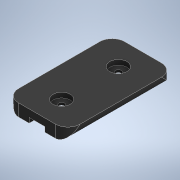
# Autodesk Inventor part: Gripper 5-4
Saved by Autodesk Inventor 2021 (Build 250183000, 183)
## iProperties
Created: 2022-01-10
Part Number: Gripper 5-4
Material: Generic
Document SubType Name: Modeling
Designer: Łukasz
Density: 1 g/cm^3
Appearance: Rubber - Black
Author: Łukasz
Autodesk Inventor part; units mm, degrees
ref_plane "YZ Plane" through (0, 0, 0) normal (1, 0, 0) x (0, 1, 0)
ref_plane "XZ Plane" through (0, 0, 0) normal (0, 1, 0) x (-1, 0, 0)
ref_plane "XY Plane" through (0, 0, 0) normal (0, 0, 1) x (1, 0, 0)
sketch "Sketch1" plane through (0, 0, 0) normal (0, 0, 1) x (1, 0, 0)
  line L0 (0, 2) -> (3.2, 2)
  line L1 (3.2, 2) -> (3.2, 0)
  line L2 (3.2, 0) -> (12.5, 0)
  line L3 (12.5, 0) -> (12.5, 5)
  line L4 (12.5, 5) -> (0, 5)
  line L5 (0, 0) -> (0, 5) construction
  line L6 (0, 2) -> (-3.2, 2)
  line L7 (-3.2, 2) -> (-3.2, 0)
  line L8 (-3.2, 0) -> (-12.5, 0)
  line L9 (-12.5, 0) -> (-12.5, 5)
  line L10 (-12.5, 5) -> (0, 5)
  dimension "d0" = 3.2
  dimension "d1" = 2
  dimension "d2" = 9.3
  dimension "d3" = 5
  constraints: 22 end point, 4 perpendicular, 4 symmetric about line, 1 horizontal, 1 vertical
  measures "d0" distance of L0.start L0.end
  measures "d1" distance from line of L5.start L0
  measures "d2" distance of L1.end L2.end
  measures "d3" distance of L2.end L3.end
extrude "Extrusion1" add sketch "Sketch1" along normal blind 43
sketch "Sketch2" plane through (-12.5, 5, 0) normal (0, 1, 0) x (1, 0, 0)
  circle A0 centre (12.5, -33) radius 1.25
  circle A1 centre (12.5, -10) radius 1.25
  line L0 (25, 0) -> (0, 0) projected
  line L1 (25, -43) -> (0, -43) projected
  point P0 (12.5, 0)
  dimension "d6" = 2.5
  dimension "d7" = 2.5
  dimension "d8" = 10
  dimension "d9" = 10
  constraints: 2 centre point
  measures "d6" diameter of A0
  measures "d7" diameter of A1
  measures "d8" distance from line of L0 A1.centre
  measures "d9" distance from line of L1 A0.centre
extrude "Extrusion2" cut sketch "Sketch2" against normal up to surface (3 mm away)
sketch "Sketch3" plane through (-12.5, 5, 0) normal (0, 1, 0) x (1, 0, 0)
  circle A0 centre (12.5, -33) radius 1.25 projected
  circle A1 centre (12.5, -33) radius 3.5
  circle A2 centre (12.5, -10) radius 1.25 projected
  circle A3 centre (12.5, -10) radius 3.5
  point P0 (12.5, 0)
  dimension "d12" = 7
  dimension "d13" = 7
  constraints: 2 centre point, 2 coincident
  measures "d12" diameter of A1
  measures "d13" diameter of A3
extrude "Extrusion3" cut sketch "Sketch3" against normal blind 2
fillet "Fillet1" radius 5 6 edges at (-12.5, 2.5, 0) (12.5, 2.5, 0) (12.5, 2.5, 43) (-12.5, 2.5, 43) (12.5, 0, 21.5) (-12.5, 0, 21.5)
body "Solid1"
